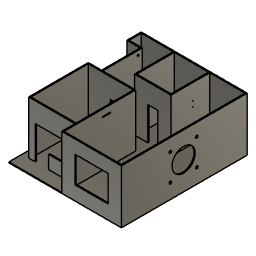
Double-room v1 (Autodesk Fusion 360 design; units mm, degrees)
Autodesk Fusion 360 part; units mm, degrees
note: some values were not read from the file. Set by a fixed rule: which sketch regions a step uses.
sketch "Sketch1" plane through (0, 0, 0) normal (0, 0, 1) x (1, 0, 0)
  line L0 (0, 100) -> (90, 100)
  line L1 (90, 100) -> (90, -90)
  line L2 (90, -90) -> (0, -90)
  line L3 (0, -90) -> (0, -70)
  line L4 (0, -70) -> (-70, -70)
  line L5 (-70, -70) -> (-70, 20)
  line L6 (-50, 20) -> (-70, 20)
  line L7 (-50, 100) -> (0, 100)
  line L8 (88.4, 98.4) -> (88.4, -88.4)
  line L9 (88.4, -88.4) -> (1.6, -88.4)
  line L10 (1.6, -88.4) -> (1.6, -68.4)
  line L11 (0, -68.4) -> (-68.4, -68.4)
  line L12 (-68.4, -68.4) -> (-68.4, 18.4)
  line L13 (-48.4, 18.4) -> (-68.4, 18.4)
  line L14 (-48.4, 20) -> (-48.4, 80)
  line L15 (0, 18.4) -> (0, -68.4)
  line L16 (1.6, -68.4) -> (1.6, 20)
  line L17 (15, 40) -> (30, 40)
  line L18 (0, 40) -> (-20, 40)
  line L19 (-20, 40) -> (-20, 98.4)
  line L20 (30, 40) -> (35, 40)
  line L21 (35, 40) -> (35, 98.4)
  line L22 (33.4, 41.6) -> (33.4, 98.4)
  line L23 (30, 41.6) -> (33.4, 41.6)
  line L24 (15, 41.6) -> (30, 41.6)
  line L25 (0, 41.6) -> (-18.4, 41.6)
  line L26 (-18.4, 41.6) -> (-18.4, 98.4)
  line L27 (-48.4, 98.4) -> (-20, 98.4)
  line L28 (-18.4, 98.4) -> (0, 98.4)
  line L29 (0, 98.4) -> (33.4, 98.4)
  line L30 (35, 98.4) -> (88.4, 98.4)
  line L31 (-35, 20) -> (-35, 18.4)
  line L32 (-20, 20) -> (-20, 18.4)
  line L33 (-48.4, 18.4) -> (-35, 18.4)
  line L34 (-20, 18.4) -> (0, 18.4)
  line L35 (1.6, 20) -> (-20, 20)
  line L36 (-35, 20) -> (-48.4, 20)
  line L37 (0, 40) -> (0, 41.6)
  line L38 (15, 41.6) -> (15, 40)
  line L39 (-50, 78.4) -> (-70, 78.4)
  line L40 (-70, 100) -> (-50, 100)
  line L41 (-48.4, 98.4) -> (-68.4, 98.4)
  line L42 (-50, 80) -> (-68.4, 80)
  line L43 (-68.4, 98.4) -> (-50, 98.4)
  line L44 (-50, 20) -> (-50, 78.4)
  line L45 (-50, 80) -> (-48.4, 80)
  line L46 (-70, 98.4) -> (-70, 100)
  line L47 (-68.4, 80) -> (-70, 80)
  line L48 (-70, 80) -> (-70, 78.4)
  line L49 (-68.4, 98.4) -> (-70, 98.4)
  dimension "d1" = 90
  dimension "d2" = 190
  dimension "d13" = 1.6
  dimension "d14" = 20
  constraint horizontal L0
  constraint perpendicular L0 L1
  constraint perpendicular L1 L2
  constraint perpendicular L2 L3
  constraint perpendicular L3 L4
  constraint perpendicular L0 L5
  constraint perpendicular L5 L6
  constraint perpendicular L0 L44
  constraint perpendicular L7 L44
  constraint perpendicular L10 L33
  constraint perpendicular L11 L15
  constraint perpendicular L16 L33
  constraint perpendicular L14 L35
  constraint perpendicular L8 L17
  constraint perpendicular L19 L27
  constraint parallel L17 L20
  constraint coincident L21.end L29
  constraint perpendicular L0 L21
  constraint collinear L27 L28
  constraint collinear L29 L30
  constraint coincident L31.start L35
  constraint perpendicular L31 L33
  constraint coincident L32.end L33
  constraint perpendicular L32 L33
  constraint collinear L33 L34
  constraint collinear L35 L36
  constraint perpendicular L17 L38
  constraint perpendicular L39 L44
  constraint perpendicular L40 L44
  constraint perpendicular L44 L45
  constraint parallel L42 L47
  constraint perpendicular L46 L49
  measures "d1" distance of L0.start L0.end
  measures "d2" distance of L0.end L1.end
  measures "d13" distance of L31.start L31.end
  measures "d14" distance of L5.end L6.start
extrude "Extrude1" add sketch "Sketch1" along normal blind 50
sketch "Sketch2" plane through (0, 0, 0) normal (0, 0, -1) x (1, 0, 0)
  line L0 (-70, -98.4) -> (-70, -100)
  line L1 (-70, -100) -> (90, -100)
  line L2 (90, -100) -> (90, 90)
  line L3 (90, 90) -> (0, 90)
  line L4 (0, 90) -> (0, 70)
  line L5 (0, 70) -> (-70, 70)
  line L6 (-70, 70) -> (-70, -20)
  line L7 (-70, -20) -> (-50, -20)
  line L8 (-50, -20) -> (-50, -78.4)
  line L9 (-50, -78.4) -> (-70, -78.4)
  line L10 (-70, -80) -> (-48.4, -80)
  line L11 (-48.4, -80) -> (-48.4, -20)
  line L12 (-48.4, -20) -> (-35, -20)
  line L13 (-35, -20) -> (-35, -18.4)
  line L14 (-35, -18.4) -> (-68.4, -18.4)
  line L15 (-68.4, -18.4) -> (-68.4, 68.4)
  line L16 (-68.4, 68.4) -> (0, 68.4)
  line L17 (0, 68.4) -> (0, -18.4)
  line L18 (0, -18.4) -> (-20, -18.4)
  line L19 (-20, -18.4) -> (-20, -20)
  line L20 (-20, -20) -> (1.6, -20)
  line L21 (1.6, -20) -> (1.6, 88.4)
  line L22 (1.6, 88.4) -> (88.4, 88.4)
  line L23 (88.4, 88.4) -> (88.4, -98.4)
  line L24 (88.4, -98.4) -> (35, -98.4)
  line L25 (35, -98.4) -> (35, -40)
  line L26 (35, -40) -> (15, -40)
  line L27 (15, -40) -> (15, -41.6)
  line L28 (15, -41.6) -> (33.4, -41.6)
  line L29 (33.4, -41.6) -> (33.4, -98.4)
  line L30 (33.4, -98.4) -> (-18.4, -98.4)
  line L31 (-18.4, -98.4) -> (-18.4, -41.6)
  line L32 (-18.4, -41.6) -> (0, -41.6)
  line L33 (0, -41.6) -> (0, -40)
  line L34 (0, -40) -> (-20, -40)
  line L35 (-20, -40) -> (-20, -98.4)
  line L36 (-20, -98.4) -> (-70, -98.4)
  line L37 (90, 90) -> (-70, 90)
  line L38 (90, -90) -> (90, 90)
  line L39 (-70, 90) -> (-80, 90)
  line L40 (-80, 90) -> (-80, -100)
  line L41 (-80, -100) -> (-70, -100)
  line L42 (-70, -78.4) -> (-70, -80)
  line L43 (90, -90) -> (90, -100)
  line L44 (88.4, -98.4) -> (-70, -98.4)
  line L45 (-70, -100) -> (90, -100)
  constraint coincident L2.end L3.start
  constraint perpendicular L6 L37
  constraint coincident L0.end L1.start
  constraint coincident L1.end L38.start
  constraint perpendicular L1 L40
  constraint perpendicular L0 L41
  constraint coincident L38.start L43.start
  constraint coincident L1.end L2.start
  constraint coincident L23.end L24.start
  constraint coincident L0.start L36.end
extrude "Extrude3" add sketch "Sketch2" along normal blind 1.2
sketch "Sketch4" plane through (0, 0, 50) normal (0, 0, 1) x (-1, 0, 0)
  line L0 (70, -98.4) -> (20, -98.4)
  line L1 (20, -98.4) -> (20, -40)
  line L2 (20, -40) -> (0, -40)
  line L3 (0, -40) -> (0, -41.6)
  line L4 (0, -41.6) -> (18.4, -41.6)
  line L5 (18.4, -41.6) -> (18.4, -98.4)
  line L6 (18.4, -98.4) -> (-33.4, -98.4)
  line L7 (-33.4, -98.4) -> (-33.4, -41.6)
  line L8 (-33.4, -41.6) -> (-15, -41.6)
  line L9 (-15, -41.6) -> (-15, -40)
  line L10 (-15, -40) -> (-35, -40)
  line L11 (-35, -40) -> (-35, -98.4)
  line L12 (-35, -98.4) -> (-88.4, -98.4)
  line L13 (-88.4, -98.4) -> (-88.4, 88.4)
  line L14 (-88.4, 88.4) -> (-1.6, 88.4)
  line L15 (-1.6, 88.4) -> (-1.6, -20)
  line L16 (-1.6, -20) -> (20, -20)
  line L17 (20, -20) -> (20, -18.4)
  line L18 (20, -18.4) -> (0, -18.4)
  line L19 (0, -18.4) -> (0, 68.4)
  line L20 (0, 68.4) -> (68.4, 68.4)
  line L21 (68.4, 68.4) -> (68.4, -18.4)
  line L22 (68.4, -18.4) -> (35, -18.4)
  line L23 (35, -18.4) -> (35, -20)
  line L24 (35, -20) -> (48.4, -20)
  line L25 (48.4, -20) -> (48.4, -80)
  line L26 (48.4, -80) -> (70, -80)
  line L27 (70, -80) -> (70, -78.4)
  line L28 (70, -78.4) -> (50, -78.4)
  line L29 (50, -78.4) -> (50, -20)
  line L30 (50, -20) -> (70, -20)
  line L31 (70, -20) -> (70, 70)
  line L32 (70, 70) -> (0, 70)
  line L33 (0, 70) -> (0, 90)
  line L34 (0, 90) -> (-90, 90)
  line L35 (-90, 90) -> (-90, -100)
  line L36 (-90, -100) -> (70, -100)
  line L37 (70, -100) -> (70, -98.4)
  line L38 (70, -100) -> (70, -78.4)
  line L39 (50, -78.4) -> (50, -20)
  line L40 (70, -20) -> (70, 70)
  line L41 (0, 70) -> (70, 70)
  line L42 (0, 70) -> (0, 90)
  line L43 (-90, 90) -> (0, 90)
  line L44 (-90, -100) -> (-90, 90)
  line L45 (48.4, -20) -> (-1.6, -20)
  line L46 (-1.6, -20) -> (-1.6, 88.4)
  line L47 (-1.6, 88.4) -> (-88.4, 88.4)
  line L48 (-88.4, 88.4) -> (-88.4, -98.4)
  line L49 (-88.4, -98.4) -> (-35, -98.4)
  line L50 (-35, -98.4) -> (-35, -40)
  line L51 (-35, -40) -> (20, -40)
  line L52 (20, -40) -> (20, -98.4)
  line L53 (-33.4, -41.6) -> (18.4, -41.6)
  line L54 (18.4, -98.4) -> (18.4, -43.3383)
  line L55 (18.4, -98.4) -> (-33.4, -98.4)
  line L56 (-33.4, -41.6) -> (-33.4, -98.4)
  line L57 (70, -78.4) -> (50, -78.4)
  line L58 (48.4, -80) -> (48.4, -20)
  line L59 (70, -20) -> (50, -20)
  line L60 (68.4, -18.4) -> (0, -18.4)
  line L61 (0, -18.4) -> (0, 68.4)
  line L62 (68.4, 68.4) -> (0, 68.4)
  line L63 (68.4, 68.4) -> (68.4, -18.4)
  line L64 (18.4, -43.3383) -> (18.4, -43)
  line L65 (18.4, -41.6) -> (18.4, -43.3383)
  line L66 (70, -100) -> (-90, -100)
  line L67 (20, -98.4) -> (68.4, -98.4)
  line L68 (48.4, -80) -> (68.4, -80)
  line L69 (70, -78.4) -> (68.4, -78.4)
  line L70 (68.4, -80) -> (68.4, -98.4)
  dimension "d18" = 1.6
  constraint coincident L36.end L37.start
  constraint coincident L27.end L28.start
  constraint coincident L28.end L29.start
  constraint coincident L29.end L30.start
  constraint coincident L30.end L31.start
  constraint coincident L31.end L32.start
  constraint coincident L32.end L33.start
  constraint coincident L33.end L34.start
  constraint coincident L34.end L35.start
  constraint coincident L35.end L36.start
  constraint coincident L24.end L25.start
  constraint coincident L15.end L16.start
  constraint coincident L14.end L15.start
  constraint coincident L13.end L14.start
  constraint coincident L12.end L13.start
  constraint coincident L11.end L12.start
  constraint coincident L10.end L11.start
  constraint coincident L1.end L2.start
  constraint coincident L0.end L1.start
  constraint coincident L7.end L8.start
  constraint coincident L4.end L5.start
  constraint coincident L5.end L6.start
  constraint coincident L5 L54.end
  constraint perpendicular L53 L54
  constraint coincident L6.end L7.start
  constraint coincident L25.end L26.start
  constraint coincident L21.end L22.start
  constraint coincident L18.end L19.start
  constraint coincident L19.end L20.start
  constraint coincident L20.end L21.start
  constraint coincident L5 L64.end
  constraint parallel L5 L64
  constraint perpendicular L27 L69
  constraint perpendicular L67 L70
  measures "d18" distance of L27.end L69.end
extrude "Extrude4" add sketch "Sketch4" against normal blind 10 contours L0 L1 L2 L3 L4 L5 L6 L7 L8 L9 L10 L11 L12 L13 L14 L15 L16 L17 L18 L19 L20 L21 L22 L23 L24 L25 L26 L27 L28 L29 L30 L31 L32 L33 L34 L35 L36 L37 L38 L39 L40 L41 L42 L43 L44 L45 L46 L47 L48 L49 L50 L51 L52 L53 L54 L55 L56 L57 L58 L59 L60 L61 L62 L63 L64 L65 L66 L67 L68 L69 | L0 L26 L38 L70 | L3 L9 L51 L53 | L17 L23 L45 L60
extrude "Extrude5" add 1 faces at (0, 99.4667, 50) along direction (0, 0, 1) blind 20
sketch "Sketch5" plane through (-50, 0, 0) normal (-1, 0, 0) x (0, -1, 0)
  line L0 (-78.4, 70) -> (-78.4, 0)
  line L1 (-78.4, 0) -> (-20, 0)
  line L2 (-20, 0) -> (-20, 70)
  line L3 (-20, 70) -> (-78.4, 70)
  line L4 (-20, 0) -> (-78.4, 0)
  line L5 (-21.0521, 0.5246) -> (-77.0521, 0.5246)
  line L6 (-77.0521, 0.5246) -> (-77.0521, 76.5246)
  line L7 (-21.0521, 0.5246) -> (-21.0521, 76.5246)
  line L8 (-21.0521, 76.5246) -> (-77.0521, 76.5246)
  line L9 (-49.0521, 0.5246) -> (-24.3521, 0.5246)
  line L10 (-37.2151, 35.9513) -> (-37.2151, 35.1419)
  line L11 (-21.0521, 38.5246) -> (-21.0521, 3.7246)
  circle A0 centre (-24.3521, 3.7246) radius 1.5
  line L12 (-49.0521, 0.5246) -> (-49.0521, 1.1)
  line L13 (-21.0521, 38.5246) -> (-23.2541, 38.5246)
  circle A1 centre (-73.7521, 3.7246) radius 1.5
  circle A2 centre (-24.3521, 73.3246) radius 1.5
  circle A3 centre (-73.7521, 73.3246) radius 1.5
  dimension "d23" = 56
  dimension "d24" = 76
  dimension "d25" = 76
  dimension "d26" = 24.7
  dimension "d27" = 34.8
  dimension "d28" = 3
  constraint coincident L1.end L2.start
  constraint coincident L0.end L1.start
  constraint perpendicular L2 L5
  constraint perpendicular L5 L6
  constraint perpendicular L5 L7
  constraint midpoint L5 L9.start
  constraint parallel L5 L9
  constraint perpendicular L8 L10
  constraint midpoint L7 L11.start
  constraint parallel L7 L11
  constraint perpendicular L5 L12
  constraint perpendicular L11 L13
  constraint symmetric A0 L12 A1
  constraint symmetric A0 L13 A2
  constraint symmetric L13 A1 A3
  measures "d23" distance of L5.start L5.end
  measures "d24" distance of L5.end L6.end
  measures "d25" distance of L5.start L7.end
  measures "d26" distance of L9.start L9.end
  measures "d27" distance of L11.start L11.end
  measures "d28" diameter of A0
extrude "Extrude6" add 1 faces at (0, 99.4667, 70) along direction (0, 0, 1) blind 10
extrude "Extrude7" cut sketch "Sketch5" against normal blind 15 contours A0 | A1 | A2 | A3
extrude "Extrude8" cut 3 faces at (-69.4667, 92.2667, 40) (-30, 19.4667, 40) (10, 40.5333, 40) along direction (0, 0, 1) blind 10
sketch "Sketch6" plane through (0, -70, 0) normal (0, -1, 0) x (1, 0, 0)
  line L0 (-70, 80) -> (-70, 0)
  line L1 (-70, 0) -> (0, 0)
  line L2 (0, 0) -> (0, 80)
  line L3 (0, 80) -> (-70, 80)
  line L4 (-60, 0) -> (-40, 0)
  line L5 (-40, 0) -> (-40, 20)
  line L6 (-40, 50) -> (-60, 50)
  line L7 (-60, 50) -> (-60, 0)
  line L8 (-40, 50) -> (-15, 50)
  line L9 (-15, 50) -> (-15, 20)
  line L10 (-15, 20) -> (-40, 20)
  constraint horizontal L4
  constraint vertical L5
  constraint horizontal L6
  constraint vertical L7
  constraint coincident L1 L4.start
  constraint horizontal L8
  constraint vertical L9
  constraint horizontal L10
extrude "Extrude9" cut sketch "Sketch6" against normal blind 10 contours L1 L4 L5 L6 L7 L8 L9 L10
sketch "Sketch7" plane through (0, -90, 0) normal (0, -1, 0) x (1, 0, 0)
  line L0 (0, 80) -> (0, 0)
  line L1 (0, 0) -> (-80, 0)
  line L2 (-80, 0) -> (-80, -1.2)
  line L3 (-80, -1.2) -> (90, -1.2)
  line L4 (90, -1.2) -> (90, 80)
  line L5 (90, 80) -> (0, 80)
  line L6 (20, 60) -> (70, 60)
  line L7 (70, 60) -> (70, 20)
  line L8 (70, 20) -> (20, 20)
  line L9 (20, 20) -> (20, 60)
  constraint horizontal L6
  constraint vertical L7
  constraint horizontal L8
  constraint vertical L9
extrude "Extrude10" cut sketch "Sketch7" against normal blind 15 contours L6 L7 L8 L9
sketch "Sketch8" plane through (0, 78.4, 0) normal (0, -1, 0) x (1, 0, 0)
  line L0 (-70, 80) -> (-70, 0)
  line L1 (-70, 0) -> (-50, 0)
  line L2 (-50, 0) -> (-50, 80)
  line L3 (-50, 80) -> (-70, 80)
  line L4 (-50, 70) -> (-60, 70)
  line L5 (-60, 70) -> (-60, 5)
  line L6 (-60, 5) -> (-50, 5)
  line L7 (-50, 5) -> (-50, 70)
  constraint horizontal L4
  constraint vertical L5
  constraint horizontal L6
  constraint vertical L7
  constraint coincident L2 L4.start
extrude "Extrude11" cut sketch "Sketch8" against normal blind 5 contours L2 L4 L5 L6 L7
sketch "Sketch9" plane through (88.4, 0, 0) normal (-1, 0, 0) x (0, -1, 0)
  line L0 (-98.4, 80) -> (-98.4, 0)
  line L1 (-98.4, 0) -> (88.4, 0)
  line L2 (88.4, 0) -> (88.4, 80)
  line L3 (88.4, 80) -> (-98.4, 80)
  line L4 (16.025, 60.9625) -> (-23.975, 60.9625)
  line L5 (-23.975, 60.9625) -> (-23.975, 20.9625)
  line L6 (-23.975, 20.9625) -> (16.025, 20.9625)
  line L7 (16.025, 20.9625) -> (16.025, 60.9625)
  circle A0 centre (16.025, 60.9625) radius 2
  circle A1 centre (-23.975, 60.9625) radius 2
  circle A2 centre (16.025, 20.9625) radius 2
  circle A3 centre (-23.975, 20.9625) radius 2
  circle A4 centre (-3.975, 40.9625) radius 17.5
  dimension "d41" = 4
  dimension "d42" = 4
  dimension "d43" = 4
  dimension "d44" = 4
  dimension "d45" = 35
  constraint horizontal L4
  constraint vertical L5
  constraint horizontal L6
  constraint vertical L7
  constraint coincident L4.start L7.end
  constraint coincident L4.end L5.start
  constraint coincident L6.end L7.start
  constraint coincident L5.end L6.start
  measures "d41" diameter of A0
  measures "d42" diameter of A1
  measures "d43" diameter of A2
  measures "d44" diameter of A3
  measures "d45" diameter of A4
extrude "Extrude12" cut sketch "Sketch9" against normal blind 9 contours L4 L5 A1 | L4 L5 A1 | L4 L7 A0 | L4 L7 A0 | L5 L6 A3 | L5 L6 A3 | L6 L7 A2 | L6 L7 A2 | A4
sketch "Sketch10" plane through (35, 0, 0) normal (1, 0, 0) x (0, 1, 0)
  line L0 (40, 80) -> (40, 0)
  line L1 (40, 0) -> (98.4, 0)
  line L2 (98.4, 0) -> (98.4, 80)
  line L3 (98.4, 80) -> (40, 80)
  circle A0 centre (73, 55.8) radius 0.5
  circle A1 centre (72.9634, 48.2002) radius 0.5
  dimension "d49" = 1
  dimension "d50" = 1
  measures "d49" diameter of A0
  measures "d50" diameter of A1
extrude "Extrude13" cut sketch "Sketch10" against normal blind 2 contours A0 | A1
sketch "Sketch11" plane through (1.6, 0, 0) normal (1, 0, 0) x (0, 1, 0)
  line L0 (-88.4, 80) -> (-88.4, 0)
  line L1 (-88.4, 0) -> (20, 0)
  line L2 (20, 0) -> (20, 80)
  line L3 (20, 80) -> (-88.4, 80)
  line L4 (-30, 70) -> (-18, 70)
  line L5 (-18, 70) -> (-18, 69)
  line L6 (-30, 70) -> (-30, 69)
  line L7 (-30, 69) -> (-18, 69)
  dimension "d53" = 12
  dimension "d54" = 1
  dimension "d55" = 1
  constraint horizontal L4
  constraint vertical L5
  constraint vertical L6
  measures "d53" distance of L4.start L4.end
  measures "d54" distance of L4.end L5.end
  measures "d55" distance of L4.start L6.end
extrude "Extrude14" cut sketch "Sketch11" against normal blind 20 contours L4 L5 L6 L7
extrude "Extrude2" add sketch "Sketch2" along normal blind 1.2 contours L0 L4 L5 L6 L7 L8 L9 L10 L11 L12 L13 L14 L15 L16 L17 L18 L19 L20 L21 L22 L23 L24 L25 L26 L27 L28 L29 L30 L31 L32 L33 L34 L35 L36 L37 L39 L40 L41 L42 L44
sketch "Sketch3" plane through (-50, 0, 0) normal (-1, 0, 0) x (0, -1, 0)
  line L0 (-78.4, 0) -> (-20, 0)
  line L1 (-20, 0) -> (-20, 50)
  line L2 (-20, 50) -> (-78.4, 50)
  line L3 (-78.4, 50) -> (-78.4, 0)
